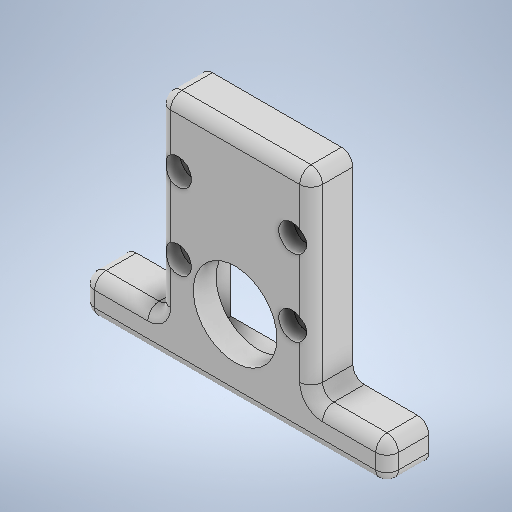
# Autodesk Inventor part: stopper_motor_bracket_cover
Saved by Autodesk Inventor 2026.1 (Build 301233000, 233)
## iProperties
Created: 2026-05-22
Part Number: stopper_motor_bracket_cover
Material: Generic
Document SubType Name: Modeling
Designer: chris
Density: 1 g/cm^3
Appearance: Default
Author: chris
Autodesk Inventor part; units mm, degrees
ref_plane "YZ Plane" through (0, 0, 0) normal (1, 0, 0) x (0, 1, 0)
ref_plane "XZ Plane" through (0, 0, 0) normal (0, 1, 0) x (-1, 0, 0)
ref_plane "XY Plane" through (0, 0, 0) normal (0, 0, 1) x (1, 0, 0)
sketch "Sketch1" plane through (0, 0, 0) normal (0, 0, 1) x (1, 0, 0)
  line L0 (-40, -40) -> (40, -40)
  line L1 (40, -40) -> (40, 40)
  line L2 (40, 40) -> (-40, 40)
  line L3 (-40, 40) -> (-40, -40)
  line L4 (-40, -40) -> (40, 40) construction
  line L5 (40, -40) -> (-40, 40) construction
  point P0 (0, 0)
  dimension "d0" = 80
  dimension "d1" = 80
  constraints: 12 end point, 2 midpoint, 2 parallel, 1 horizontal, 1 perpendicular
  measures "d0" distance of L2.end L1.end
  measures "d1" distance of L1.end L0.end
extrude "Extrusion1" add sketch "Sketch1" along normal blind 6
sketch "Sketch2" plane through (0, 0, 0) normal (0, 0, -1) x (-1, 0, 0)
  arc A0 (37, -21.1) -> (40, -18.1) centre (37, -18.1) ccw projected
  line L0 (37, -21.1) -> (-37, -21.1) projected
  arc A1 (-40, -18.1) -> (-37, -21.1) centre (-37, -18.1) ccw projected
  line L1 (-40, -14.1) -> (-40, -18.1) projected
  arc A2 (-37, -11.1) -> (-40, -14.1) centre (-37, -14.1) ccw projected
  line L2 (-23, -11.1) -> (-37, -11.1) projected
  arc A3 (-23, -11.1) -> (-20, -8.1) centre (-23, -8.1) ccw projected
  line L3 (-20, -8.1) -> (-20, 37) projected
  arc A4 (-17, 40) -> (-20, 37) centre (-17, 37) ccw projected
  line L4 (17, 40) -> (-17, 40) projected
  arc A5 (20, 37) -> (17, 40) centre (17, 37) ccw projected
  line L5 (20, 37) -> (20, -8.1) projected
  arc A6 (20, -8.1) -> (23, -11.1) centre (23, -8.1) ccw projected
  line L6 (37, -11.1) -> (23, -11.1) projected
  arc A7 (40, -14.1) -> (37, -11.1) centre (37, -14.1) ccw projected
  line L7 (40, -14.1) -> (40, -18.1) projected
  circle A8 centre (15, 3.9) radius 2 projected
  circle A9 centre (-15, 3.9) radius 2 projected
  circle A10 centre (15, 23.9) radius 2 projected
  circle A11 centre (-15, 23.9) radius 2 projected
  line L8 (12.1, 32) -> (12.1, -13.1) projected
  line L9 (-12.1, 32) -> (12.1, 32) projected
  line L10 (-12.1, -13.1) -> (-12.1, 32) projected
  line L11 (12.1, -13.1) -> (-12.1, -13.1) projected
  circle A12 centre (0, -1.1) radius 7.5 projected
  line L12 (-40, -40) -> (40, -40)
  line L13 (40, -40) -> (40, 40)
  line L14 (40, 40) -> (-40, 40)
  line L15 (-40, 40) -> (-40, -40)
  line L16 (-40, -40) -> (40, 40) construction
  line L17 (40, -40) -> (-40, 40) construction
  line L18 (-40, 40) -> (40, 40) projected
  line L19 (40, 40) -> (40, -40) projected
  line L20 (-40, -40) -> (-40, 40) projected
  line L21 (40, -40) -> (-40, -40) projected
  point P0 (0, 0)
  point P1 (0, 0)
  point P2 (-40, -18.1)
  constraints: 12 end point, 4 collinear, 2 midpoint, 2 parallel, 1 horizontal, 1 perpendicular
extrude "Extrusion2" cut sketch "Sketch2" against normal blind 6 contours A0 L13 L12 L15 A1 L0 | A7 L6 A6 L5 A5 L14 L13 | L15 L14 A4 L3 A3 L2 A2 | A8 | A9 | A10 | A11 | A12
sketch "Sketch3" plane through (0, 0, 0) normal (0, 0, -1) x (-1, 0, 0)
  arc A0 (37, -21.1) -> (40, -18.1) centre (37, -18.1) ccw projected
  line L0 (37, -21.1) -> (-37, -21.1) projected
  arc A1 (-40, -18.1) -> (-37, -21.1) centre (-37, -18.1) ccw projected
  line L1 (-40, -14.1) -> (-40, -18.1) projected
  arc A2 (-37, -11.1) -> (-40, -14.1) centre (-37, -14.1) ccw projected
  line L2 (-23, -11.1) -> (-37, -11.1) projected
  arc A3 (-23, -11.1) -> (-20, -8.1) centre (-23, -8.1) ccw projected
  line L3 (-20, -8.1) -> (-20, 37) projected
  arc A4 (-17, 40) -> (-20, 37) centre (-17, 37) ccw projected
  line L4 (17, 40) -> (-17, 40) projected
  arc A5 (20, 37) -> (17, 40) centre (17, 37) ccw projected
  line L5 (20, 37) -> (20, -8.1) projected
  arc A6 (20, -8.1) -> (23, -11.1) centre (23, -8.1) ccw projected
  line L6 (37, -11.1) -> (23, -11.1) projected
  arc A7 (40, -14.1) -> (37, -11.1) centre (37, -14.1) ccw projected
  line L7 (40, -14.1) -> (40, -18.1) projected
  circle A8 centre (15, 3.9) radius 2 projected
  circle A9 centre (-15, 3.9) radius 2 projected
  circle A10 centre (15, 23.9) radius 2 projected
  circle A11 centre (-15, 23.9) radius 2 projected
  line L8 (12.1, 32) -> (12.1, -13.1) projected
  line L9 (-12.1, 32) -> (12.1, 32) projected
  line L10 (-12.1, -13.1) -> (-12.1, 32) projected
  line L11 (12.1, -13.1) -> (-12.1, -13.1) projected
  point P0 (0, 0)
extrude "Extrusion3" add sketch "Sketch3" along normal blind 5
sketch "Sketch4" plane through (0, 0, 6) normal (0, 0, 1) x (1, 0, 0)
  circle A0 centre (0, -1.1) radius 7.5 projected
  circle A1 centre (0, -1.1) radius 11
  point P0 (0, 0)
  dimension "d8" = 22
  constraints: 1 centre point, 1 coincident
  measures "d8" diameter of A1
extrude "Extrusion4" cut sketch "Sketch4" against normal through all
fillet "Fillet1" radius 3 16 edges at (-19.1213, 39.1213, 6) (-20, 14.45, 6) (-20.8787, -10.2213, 6) (-30, -11.1, 6) (-39.1213, -11.9787, 6) (-40, -16.1, 6) (-39.1213, -20.2213, 6) (0, -21.1, 6) (39.1213, -20.2213, 6) (40, -16.1, 6) (39.1213, -11.9787, 6) (30, -11.1, 6) (20.8787, -10.2213, 6) (20, 14.45, 6) (19.1213, 39.1213, 6) (0, 40, 6)
sketch "Sketch5" plane through (0, 0, 6) normal (0, 0, 1) x (1, 0, 0)
  circle A0 centre (-15, 23.9) radius 2 projected
  line L0 (-17, 3.9) -> (-17, 23.9) projected
  circle A1 centre (-15, 3.9) radius 2 projected
  line L1 (-17, -8.1) -> (-17, 3.9) projected
  arc A2 (-23, -14.1) -> (-17, -8.1) centre (-23, -8.1) ccw projected
  line L2 (-37, -14.1) -> (-23, -14.1) projected
  line L3 (-37, -18.1) -> (-37, -14.1) projected
  line L4 (37, -18.1) -> (-37, -18.1) projected
  line L5 (37, -14.1) -> (37, -18.1) projected
  line L6 (23, -14.1) -> (37, -14.1) projected
  arc A3 (17, -8.1) -> (23, -14.1) centre (23, -8.1) ccw projected
  line L7 (17, 3.9) -> (17, -8.1) projected
  circle A4 centre (15, 3.9) radius 2 projected
  line L8 (17, 23.9) -> (17, 3.9) projected
  circle A5 centre (15, 23.9) radius 2 projected
  line L9 (17, 37) -> (17, 23.9) projected
  line L10 (-17, 37) -> (17, 37) projected
  line L11 (-17, 23.9) -> (-17, 37) projected
  circle A6 centre (0, -1.1) radius 11 projected
  circle A7 centre (-15, 23.9) radius 3.5
  circle A8 centre (15, 23.9) radius 3.5
  circle A9 centre (-15, 3.9) radius 3.5
  circle A10 centre (15, 3.9) radius 3.5
  point P0 (0, 0)
  dimension "d12" = 7
  dimension "d13" = 7
  dimension "d14" = 7
  dimension "d15" = 7
  constraints: 4 centre point, 4 coincident, 4 horizontal alignment
  measures "d12" diameter of A7
  measures "d13" diameter of A8
  measures "d14" diameter of A9
  measures "d15" diameter of A10
extrude "Extrusion5" cut sketch "Sketch5" against normal blind 4 contours L11 A7 L0 | L0 A7 L11 | A9 L1 L0 | L0 L1 A9 | A8 L8 L9 | L9 L8 A8 | A10 L7 L8 | L8 L7 A10
body "Solid1"
